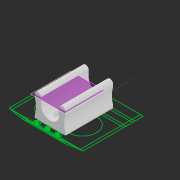
# Autodesk Inventor part: ironHolder
Saved by Autodesk Inventor 2020.3 (Build 243373010, 373A)
## iProperties
Created: 2021-04-27
Part Number: ironHolder
Material: Generic
Document SubType Name: Modeling
Designer: Melvin Strobl
Density: 1 g/cm^3
Appearance: Default
Author: Melvin Strobl
Autodesk Inventor part; units mm, degrees
ref_plane "YZ Plane" through (0, 0, 0) normal (1, 0, 0) x (0, 1, 0)
ref_plane "XZ Plane" through (0, 0, 0) normal (0, 1, 0) x (-1, 0, 0)
ref_plane "XY Plane" through (0, 0, 0) normal (0, 0, 1) x (1, 0, 0)
derived "body.ipt"
sketch "Sketch1" plane through (0, 0, 0) normal (0, 1, 0) x (-1, 0, 0)
  line L0 (0, 0) -> (53, 0)
  line L1 (53, 0) -> (53, -43)
  line L2 (0, -43) -> (0, 0)
  circle A0 centre (26.5, -33) radius 2.25
  line L3 (26.5, -65) -> (26.5, 0) construction
  line L4 (41.5, 0) -> (11.5, 0)
  line L5 (11.5, 0) -> (11.5, 2)
  line L6 (11.5, 2) -> (41.5, 2)
  line L7 (41.5, 2) -> (41.5, 0)
  circle A1 centre (34, -1) radius 2
  circle A2 centre (19, -1) radius 2
  line L8 (41.5, -1) -> (11.5, -1) construction
  line L9 (51, -43) -> (51, 0)
  line L10 (51, 0) -> (2, 0)
  line L11 (2, 0) -> (2, -43)
  line L12 (40.25, 1.25) -> (12.75, 1.25)
  line L13 (12.75, 1.25) -> (12.75, 0.75)
  line L14 (12.75, 0.75) -> (40.25, 0.75)
  line L15 (40.25, 0.75) -> (40.25, 1.25)
  line L16 (40.25, 1.25) -> (40.25, 0)
  line L17 (12.75, 1.25) -> (12.75, 0)
  line L18 (53, -43) -> (0, -43)
  circle A3 centre (26.5, -33) radius 4
  line L19 (27.75, -43) -> (28.25, -43)
  line L20 (0, -37) -> (53, -37)
  line L21 (0, -29) -> (53, -29)
  line L22 (0, -30.75) -> (53, -30.75)
  line L23 (53, -30.75) -> (53, -35.25)
  line L24 (53, -35.25) -> (0, -35.25)
  line L25 (0, -35.25) -> (0, -30.75)
  line L26 (24.4215, -36.6) -> (22.3431, -33)
  line L27 (22.3431, -33) -> (24.4215, -29.4)
  line L28 (24.4215, -29.4) -> (28.5785, -29.4)
  line L29 (28.5785, -29.4) -> (30.6569, -33)
  line L30 (30.6569, -33) -> (28.5785, -36.6)
  line L31 (28.5785, -36.6) -> (24.4215, -36.6)
  line L32 (36.5, -16) -> (16.5, -16) construction
  line L33 (36.5, -6) -> (16.5, -6)
  line L34 (16.5, -26) -> (36.5, -26)
  arc A4 (36.5, -26) -> (36.5, -6) centre (36.5, -16) ccw
  arc A5 (16.5, -6) -> (16.5, -26) centre (16.5, -16) ccw
  line L35 (41.5, 2) -> (53, 0)
  line L36 (11.5, 2) -> (0, 0)
  line L37 (12.75, 0.75) -> (2, 0)
  line L38 (40.25, 0.75) -> (51, 0)
  line L39 (19, -3) -> (34, -3)
  circle A6 centre (26.5, -1) radius 1.5
  circle A7 centre (26.5, -22) radius 1.6
  circle A8 centre (26.5, -10) radius 1.6
  point P0 (26.5, -16)
sketch "Sketch2" plane through (0, 0, 0) normal (0, 1, 0) x (-1, 0, 0)
  circle A0 centre (26.5, -22) radius 1.6 projected
  line L0 (36.5, -16) -> (16.5, -16) construction
  line L1 (26.5, -65) -> (26.5, 0) construction
  circle A1 centre (26.5, -10) radius 1.6 projected
  line L2 (11.5, 2) -> (41.5, 2) projected
  line L3 (53, -43) -> (0, -43) projected
  line L4 (33, -3) -> (20, -3)
  line L5 (20, -3) -> (20, -29)
  line L6 (33, -29) -> (33, -3)
  line L7 (33, -3) -> (20, -29) construction
  line L8 (20, -3) -> (33, -29) construction
  line L9 (37.5, -3) -> (15.5, -3)
  line L10 (15.5, -3) -> (15.5, -29)
  line L11 (37.5, -29) -> (37.5, -3)
  line L12 (37.5, -3) -> (15.5, -29) construction
  line L13 (15.5, -3) -> (37.5, -29) construction
  line L14 (26.5, -25.3486) -> (23.6, -23.6743)
  line L15 (23.6, -23.6743) -> (23.6, -20.3257)
  line L16 (23.6, -20.3257) -> (26.5, -18.6514)
  line L17 (26.5, -18.6514) -> (29.4, -20.3257)
  line L18 (29.4, -20.3257) -> (29.4, -23.6743)
  line L19 (29.4, -23.6743) -> (26.5, -25.3486)
  line L20 (26.5, -13.3486) -> (23.6, -11.6743)
  line L21 (23.6, -11.6743) -> (23.6, -8.3257)
  line L22 (23.6, -8.3257) -> (26.5, -6.6514)
  line L23 (26.5, -6.6514) -> (29.4, -8.3257)
  line L24 (29.4, -8.3257) -> (29.4, -11.6743)
  line L25 (29.4, -11.6743) -> (26.5, -13.3486)
  line L26 (33, -29) -> (33, -37.0625)
  line L27 (33, -37.0625) -> (37.5, -37.0625)
  line L28 (37.5, -37.0625) -> (37.5, -29)
  line L29 (15.5, -29) -> (15.5, -37.0625)
  line L30 (15.5, -37.0625) -> (20, -37.0625)
  line L31 (20, -37.0625) -> (20, -29)
  line L32 (20, -29) -> (20.1756, -29)
  line L33 (23.6, -28.5) -> (26.5, -28.5)
  line L34 (32.8244, -29) -> (33, -29)
  line L35 (33, -37.0625) -> (20, -37.0625)
  line L36 (24.4191, -29) -> (28.5809, -29)
  line L37 (28.5809, -29) -> (28.5809, -37.0625)
  line L38 (28.5809, -37.0625) -> (24.4191, -37.0625)
  line L39 (24.4191, -37.0625) -> (24.4191, -29)
  line L40 (24.4191, -29) -> (28.5809, -37.0625) construction
  line L41 (28.5809, -29) -> (24.4191, -37.0625) construction
  point P0 (0, 0)
  point P1 (26.5, -16)
  point P2 (20, -3)
  point P3 (33, -3)
  point P4 (26.5, -33.0312)
  dimension "d1" = 13
  dimension "d2" = 22
  dimension "d3" = 5.8
  dimension "d4" = 5.8
  constraints: 76 end point, 9 parallel, 6 midpoint, 5 point on line, 3 horizontal, 3 perpendicular, 2 coincident, 1 collinear, 31 other
  measures "d1" distance of L5.end L6.start
  measures "d2" distance of L28.end L12.end
  measures "d3" distance between parallel lines of L21 L24
  measures "d4" distance between parallel lines of L15 L18
extrude "Extrusion1" add sketch "Sketch2" along normal blind 4 contours L6 L26 L35 L37 L36 L39 L31 L5 L4 | L9 L11 L28 L27 L26 L6 | L5 L31 L30 L29 L10 L9 | L35 L39 L36 L37 | L14 L15 L16 L17 L18 L19 | L20 L21 L22 L23 L24 L25
extrude "Extrusion2" add sketch "Sketch2" along normal blind 15 contours L9 L11 L28 L27 L26 L6 | L5 L31 L30 L29 L10 L9
sketch "Sketch3" plane through (-37.5, 0, -3) normal (0, 0, 1) x (1, 0, 0)
  line L0 (4.5, 4) -> (4.5, 15) projected
  line L1 (17.5, 4) -> (17.5, 15) projected
  arc A0 (4.5, 10) -> (17.5, 10) centre (11, 10.5208) ccw
  line L2 (4.5, 4) -> (17.5, 4) projected
  line L3 (4.5, 4) -> (4.5, 15) projected
  arc A1 (4.5, 14.2891) -> (0, 15) centre (2.2996, 14.9587) ccw
  line L4 (17.5, 15) -> (22, 15) projected
  line L5 (17.5, 4) -> (17.5, 15) projected
  arc A2 (22, 15) -> (17.5, 14.2891) centre (19.7004, 14.9587) ccw
  line L6 (4.5, 4) -> (17.5, 4) projected
  line L7 (0, 0) -> (0, 15) projected
  line L8 (0, 0) -> (22, 0) projected
  line L9 (22, 0) -> (22, 15) projected
  line L10 (4.5, 4) -> (4.5, 15) projected
  line L11 (0, 15) -> (4.5, 15) projected
  line L12 (17.5, 15) -> (22, 15) projected
  line L13 (17.5, 4) -> (17.5, 15) projected
  line L14 (0, 0) -> (0, 15) projected
  arc A3 (0, 2) -> (0, 13) centre (-16.0857, 7.5) ccw
  line L15 (0, 0) -> (22, 0) construction
  line L16 (11, 0) -> (11, 10.5208) construction
  arc A4 (22, 13) -> (22, 2) centre (38.0857, 7.5) ccw
  point P0 (37.5, 0)
  point P1 (11, 4)
  point P2 (4.5, 14.2891)
  point P3 (22, 4)
  point P4 (0, 4)
  point P5 (0, 15)
  point P6 (0, 13)
  point P7 (0, 2)
  point P8 (22, 2)
  dimension "d9" = 6
  dimension "d10" = 6
  dimension "d13" = 2.3
  dimension "d14" = 2.3
  dimension "d25" = 17
  dimension "d26" = 2
  dimension "d27" = 2
  constraints: 10 point on circle, 6 point on line, 5 centre point, 3 symmetric about line, 2 end point, 1 midpoint, 1 tangent, 1 other
  measures "d9" distance of L1.start A0.end
  measures "d10" distance of L0.start A0.start
  measures "d13" radius of A1
  measures "d14" radius of A2
  measures "d25" radius of A3
  measures "d26" distance from line of L8 A3.start
  measures "d27" distance of L7.end A3.end
extrude "Extrusion3" add sketch "Sketch3" against normal blind 34.062 contours L0 A0 L2 | A0 L1 L2 | L0 L11 A1 | A2 L4 L1
fillet "Fillet1" radius 2 4 edges at (-33, 14.2891, -20.031) (-20, 14.2891, -20.031) (-33, 10, -20.031) (-20, 10, -20.031)
fillet "Fillet2" radius 2 2 edges at (-37.5, 15, -20.031) (-15.5, 15, -20.031)
ref_plane "Work Plane1" through (0, 15.25, 0) normal (0, -1, 0) x (1, 0, 0)
extrude "Extrusion4" cut sketch "Sketch2" against normal blind 14.25 from surface at 15.25 contours A0 | A1 | L35 L39 L36 L37 | L14 L15 L16 L17 L18 L19 | L20 L21 L22 L23 L24 L25
fillet "Fillet4" radius 0.4 2 edges at (-24.9, 0, -22) (-24.9, 0, -10)
fillet "Fillet5" radius 0.2 3 edges at (-15.5, 0, -20.0312) (-37.5, 0, -20.0312) (-26.5, 0, -3)
fillet "Fillet6" radius 2 6 edges at (-24.4191, 4.3409, -33.031) (-26.5, 4, -29) (-28.5809, 4.3409, -33.031) (-24.4191, 1, -33.0312) (-28.5809, 1, -33.0312) (-26.5, 1, -29)
fillet "Fillet7" radius 0.8 12 edges at (-25.0106, 4.1724, -19.5113) (-27.9894, 4.1724, -19.5113) (-29.4, 4.6803, -22) (-23.6, 4.6803, -22) (-25.0106, 4.1724, -24.4887) (-27.9894, 4.1724, -24.4887) (-25.0106, 4.1724, -7.5113) (-27.9894, 4.1724, -7.5113) (-29.4, 4.6803, -10) (-27.9894, 4.1724, -12.4887) (-25.0106, 4.1724, -12.4887) (-23.6, 4.6803, -10)
extrude "Extrusion5" cut sketch "Sketch3" against normal blind 34.063 contours A3 L7 | L9 A4
fillet "Fillet8" radius 6 6 edges at (-37.5, 13, -20.031) (-37.5, 13, -37.0622) (-37.5, 2, -20.0312) (-15.5, 13, -37.0622) (-15.5, 13, -20.031) (-15.5, 2, -20.0312)
equation "\"d4\" = d3"
equation "\"d10\" = d9"
equation "\"d14\" = d13"
body "Solid1"
